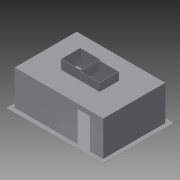
# Autodesk Inventor part: UL_NIST_Vents_Drawing
Saved by Autodesk Inventor 2013 SP2 (Build 170200200, 200)
## iProperties
Created: 2014-01-09
Part Number: UL_NIST_Vents_Drawing
Material: Generic
Document SubType Name: Modeling
Designer: mcgratta
Density: 1 g/cm^3
Author: mcgratta
Autodesk Inventor part; units mm, degrees
ref_plane "YZ Plane" through (0, 0, 0) normal (1, 0, 0) x (0, 1, 0)
ref_plane "XZ Plane" through (0, 0, 0) normal (0, 1, 0) x (-1, 0, 0)
ref_plane "XY Plane" through (0, 0, 0) normal (0, 0, 1) x (1, 0, 0)
sketch "Sketch1" plane through (0, 0, 0) normal (0, 0, 1) x (1, 0, 0)
  line L0 (-300, -300) -> (6400, -300)
  line L1 (6400, -300) -> (6400, 4600)
  line L2 (6400, 4600) -> (-300, 4600)
  line L3 (-300, 4600) -> (-300, -300)
  point P0 (0, 0)
  dimension "d0" = 300
  dimension "d3" = 6700
  dimension "d5" = 4900
  dimension "d6" = 300
  constraints: 8 end point, 2 parallel, 1 horizontal, 1 perpendicular
  measures "d0" distance from line of point (0, 0) L0
  measures "d3" distance between parallel lines of L1 L3
  measures "d5" distance between parallel lines of L2 L0
  measures "d6" distance from line of point (0, 0) L3
extrude "Extrusion1" add sketch "Sketch1" along normal blind 10
sketch "Sketch2" plane through (0, 0, 10) normal (0, 0, 1) x (1, 0, 0)
  line L0 (-300, -300) -> (6400, -300) projected
  line L1 (6400, 4600) -> (-300, 4600) projected
  line L2 (-300, 4600) -> (-300, -300) projected
  line L3 (-20, 4300) -> (0, 4300)
  line L4 (0, 4300) -> (0, 0)
  line L5 (0, 0) -> (-20, 0)
  line L6 (-20, 0) -> (-20, 4300)
  dimension "d9" = 280
  dimension "d10" = 20
  dimension "d11" = 300
  dimension "d12" = 300
  constraints: 8 end point, 2 parallel, 1 horizontal, 1 perpendicular
  measures "d9" distance between parallel lines of L6 L2
  measures "d10" distance between parallel lines of L4 L6
  measures "d11" distance from line of L1 L3.start
  measures "d12" distance from line of L0 L5.end
extrude "Extrusion2" add sketch "Sketch2" along normal blind 2400
sketch "Sketch3" plane through (0, 0, 10) normal (0, 0, 1) x (1, 0, 0)
  line L0 (0, 4300) -> (0, 0) projected
  line L1 (0, 20) -> (6100, 20)
  line L2 (6100, 20) -> (6100, 0)
  line L3 (6100, 0) -> (0, 0)
  line L4 (0, 0) -> (0, 20)
  dimension "d15" = 6100
  dimension "d17" = 20
  constraints: 8 end point, 2 parallel, 1 horizontal, 1 perpendicular, 1 point on line
  measures "d15" distance between parallel lines of L2 L4
  measures "d17" distance between parallel lines of L3 L1
extrude "Extrusion3" add sketch "Sketch3" along normal blind 2400
sketch "Sketch4" plane through (0, 0, 10) normal (0, 0, 1) x (1, 0, 0)
  line L0 (6100, 0) -> (6120, 0)
  line L1 (6120, 0) -> (6120, 4300)
  line L2 (6120, 4300) -> (6100, 4300)
  line L3 (6100, 4300) -> (6100, 0)
  point P0 (0, 0)
  dimension "d20" = 20
  dimension "d22" = 4300
  constraints: 8 end point, 2 parallel, 1 horizontal, 1 perpendicular
  measures "d20" distance between parallel lines of L1 L3
  measures "d22" vertical distance of L2.end L0.end
extrude "Extrusion4" add sketch "Sketch4" along normal blind 2400
sketch "Sketch5" plane through (0, 0, 10) normal (0, 0, 1) x (1, 0, 0)
  line L0 (0, 4300) -> (0, 20) projected
  line L1 (0, 4280) -> (6120, 4280)
  line L2 (6120, 4280) -> (6120, 4300)
  line L3 (6120, 4300) -> (0, 4300)
  line L4 (0, 4300) -> (0, 4280)
  point P0 (0, 0)
  dimension "d25" = 20
  constraints: 8 end point, 2 parallel, 1 horizontal, 1 perpendicular, 1 point on line
  measures "d25" distance between parallel lines of L3 L1
extrude "Extrusion5" add sketch "Sketch5" along normal blind 2400
sketch "Sketch6" plane through (-20, 0, 10) normal (0, -1, 0) x (1, 0, 0)
  line L0 (6140, 0) -> (0, 0) projected
  line L1 (4320, 0) -> (5220, 0)
  line L2 (5220, 0) -> (5220, 2100)
  line L3 (5220, 2100) -> (4320, 2100)
  line L4 (4320, 2100) -> (4320, 0)
  line L5 (20, 2400) -> (20, 0) projected
  point P0 (20, -10)
  dimension "d29" = 4300
  dimension "d30" = 900
  dimension "d31" = 2100
  constraints: 8 end point, 2 parallel, 1 horizontal, 1 perpendicular, 1 point on line
  measures "d29" distance between parallel lines of L4 L5
  measures "d30" distance between parallel lines of L2 L4
  measures "d31" distance from line of L3 L1.end
extrude "Extrusion6" cut sketch "Sketch6" along normal mid plane 40
sketch "Sketch7" plane through (0, 0, 10) normal (0, 0, 1) x (1, 0, 0)
  line L0 (6100, 4280) -> (0, 4280) projected
  line L1 (0, 4280) -> (0, 20) projected
  line L2 (5, 4275) -> (765, 4275)
  line L3 (765, 4275) -> (765, 3515)
  line L4 (765, 3515) -> (5, 3515)
  line L5 (5, 3515) -> (5, 4275)
  point P0 (0, 0)
  dimension "d34" = 760
  dimension "d36" = 760
  dimension "d37" = 5
  dimension "d38" = 5
  constraints: 8 end point, 2 parallel, 1 horizontal, 1 perpendicular
  measures "d34" distance between parallel lines of L3 L5
  measures "d36" distance between parallel lines of L4 L2
  measures "d37" distance between parallel lines of L2 L0
  measures "d38" distance between parallel lines of L5 L1
extrude "Extrusion7" add sketch "Sketch7" along normal blind 390
sketch "Sketch8" plane through (-20, 0, 10) normal (0, -1, 0) x (1, 0, 0)
  line L0 (0, 2400) -> (6140, 2400)
  line L1 (6140, 2400) -> (6140, 2420)
  line L2 (6140, 2420) -> (0, 2420)
  line L3 (0, 2420) -> (0, 2400)
  point P0 (20, -10)
  dimension "d41" = 20
  constraints: 8 end point, 2 parallel, 1 horizontal, 1 perpendicular
  measures "d41" distance between parallel lines of L2 L0
extrude "Extrusion8" add sketch "Sketch8" against normal blind 4300
sketch "Sketch9" plane through (-20, 0, 2430) normal (0, 0, 1) x (1, 0, 0)
  line L0 (0, 4300) -> (6140, 4300) projected
  line L1 (0, 0) -> (0, 4300) projected
  line L2 (1750, 2800) -> (3050, 2800)
  line L3 (3050, 2800) -> (3050, 1500)
  line L4 (3050, 1500) -> (1750, 1500)
  line L5 (1750, 1500) -> (1750, 2800)
  line L6 (1730, 2820) -> (3070, 2820)
  line L7 (3070, 2820) -> (3070, 1480)
  line L8 (3070, 1480) -> (1730, 1480)
  line L9 (1730, 1480) -> (1730, 2820)
  point P0 (20, 0)
  dimension "d45" = 1500
  dimension "d46" = 1300
  dimension "d47" = 1300
  dimension "d48" = 1750
  dimension "d49" = 20
  dimension "d50" = 20
  dimension "d51" = 20
  dimension "d52" = 20
  constraints: 16 end point, 4 parallel, 2 horizontal, 2 perpendicular
  measures "d45" distance between parallel lines of L0 L2
  measures "d46" distance between parallel lines of L4 L2
  measures "d47" distance between parallel lines of L3 L5
  measures "d48" distance between parallel lines of L5 L1
  measures "d49" distance between parallel lines of L2 L6
  measures "d50" distance between parallel lines of L5 L9
  measures "d51" distance between parallel lines of L4 L8
  measures "d52" distance between parallel lines of L7 L3
extrude "Extrusion9" add sketch "Sketch9" along normal blind 640
sketch "Sketch10" plane through (1730, 2800, 2430) normal (0, 0, 1) x (1, 0, 0)
  line L0 (1300, -1300) -> (1300, 0) projected
  line L1 (1300, 0) -> (0, 0) projected
  line L2 (0, 0) -> (1300, 0)
  line L3 (1300, 0) -> (1300, -1300)
  line L4 (1300, -1300) -> (0, -1300)
  line L5 (0, -1300) -> (0, 0)
  point P0 (-1730, -2800)
  constraints: 8 end point, 2 parallel, 1 horizontal, 1 perpendicular
extrude "Extrusion10" cut sketch "Sketch10" against normal blind 40
sketch "Sketch11" plane through (-20, 0, 2430) normal (0, 0, 1) x (1, 0, 0)
  line L0 (3070, 2820) -> (3070, 1480) projected
  line L1 (3070, 2820) -> (4410, 2820)
  line L2 (4410, 2820) -> (4410, 1480)
  line L3 (4410, 1480) -> (3070, 1480)
  line L4 (3070, 1480) -> (3070, 2820)
  line L5 (3090, 2800) -> (4390, 2800)
  line L6 (4390, 2800) -> (4390, 1500)
  line L7 (4390, 1500) -> (3090, 1500)
  line L8 (3090, 1500) -> (3090, 2800)
  point P0 (20, 0)
  dimension "d57" = 1340
  dimension "d59" = 20
  dimension "d60" = 20
  dimension "d61" = 20
  dimension "d62" = 20
  constraints: 16 end point, 4 parallel, 2 horizontal, 2 perpendicular
  measures "d57" distance between parallel lines of L2 L4
  measures "d59" distance between parallel lines of L8 L0
  measures "d60" distance between parallel lines of L5 L1
  measures "d61" distance between parallel lines of L3 L7
  measures "d62" distance between parallel lines of L2 L6
extrude "Extrusion11" add sketch "Sketch11" along normal blind 550
sketch "Sketch12" plane through (3070, 2800, 2430) normal (0, 0, 1) x (1, 0, 0)
  line L0 (1300, -1300) -> (1300, 0) projected
  line L1 (1300, 0) -> (0, 0) projected
  line L2 (0, 0) -> (1300, 0)
  line L3 (1300, 0) -> (1300, -1300)
  line L4 (1300, -1300) -> (0, -1300)
  line L5 (0, -1300) -> (0, 0)
  point P0 (-3070, -2800)
  constraints: 8 end point, 2 parallel, 1 horizontal, 1 perpendicular
extrude "Extrusion12" cut sketch "Sketch12" against normal blind 40
sketch "Sketch14" plane through (-20, 0, 10) normal (-1, 0, 0) x (0, 0, 1)
  line L0 (0, 0) -> (0, 4300) projected
  line L1 (0, 4300) -> (2420, 4300) projected
  arc A0 (0, 2458.5455) -> (1841.4545, 4300) centre (0, 4300) ccw
  line L2 (1841.4545, 4300) -> (0, 4300)
  line L3 (0, 4300) -> (0, 2458.5455)
  point P0 (-10, 0)
  constraints: 4 end point, 2 collinear, 2 point on circle, 1 centre point, 1 coincident, 1 point on line
extrude "Extrusion14" cut sketch "Sketch14" along normal mid plane 40
body "Solid1"
